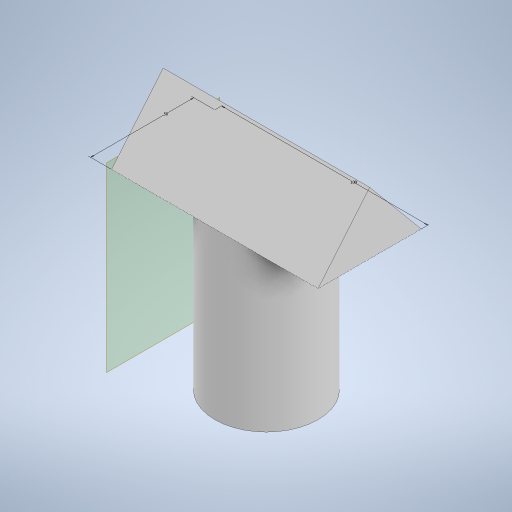
# Autodesk Inventor part: rotator_flat
Saved by Autodesk Inventor 2023.1 (Build 271208000, 208)
## iProperties
Created: 2022-10-07
Part Number: rotator_flat
Material: Generic
Document SubType Name: Modeling
Designer: swang
Density: 1 g/cm^3
Appearance: Default
Author: swang
Autodesk Inventor part; units mm, degrees
ref_plane "YZ Plane" through (0, 0, 0) normal (1, 0, 0) x (0, 1, 0)
ref_plane "XZ Plane" through (0, 0, 0) normal (0, 1, 0) x (-1, 0, 0)
ref_plane "XY Plane" through (0, 0, 0) normal (0, 0, 1) x (1, 0, 0)
sketch "Sketch1" plane through (0, 0, 0) normal (0, 1, 0) x (-1, 0, 0)
  circle A0 centre (0, 0) radius 25
  dimension "d0" = 50
  constraints: 1 centre point, 1 coincident
  measures "d0" diameter of A0
extrude "Extrusion1" add sketch "Sketch1" along normal blind 80
sketch "Sketch3" plane through (0, 80, 0) normal (0, 1, 0) x (1, 0, 0)
  line L0 (-50, -25) -> (50, -25) construction
  line L1 (50, -25) -> (50, 25) construction
  line L2 (50, 25) -> (-50, 25) construction
  line L3 (-50, 25) -> (-50, -25) construction
  line L4 (-50, -25) -> (50, 25) construction
  line L5 (50, -25) -> (-50, 25) construction
  point P0 (0, 0)
  dimension "d7" = 100
  dimension "d8" = 50
  constraints: 12 end point, 2 midpoint, 2 parallel, 1 horizontal, 1 perpendicular
  measures "d7" distance of L1.end L2.end
  measures "d8" distance of L2.end L0.start
ref_plane "Work Plane2" through (-50, 80, -25) normal (-1, 0, 0) x (0, 0, 1)
sketch "Sketch5" plane through (-50, 80, -25) normal (-1, 0, 0) x (0, 0, 1)
  line L0 (50, 0) -> (0, 0) projected
  line L1 (50, 0) -> (0, 0)
  line L2 (25, 0) -> (25, 30) construction
  line L3 (25, 30) -> (50, 0)
  line L4 (25, 30) -> (0, 0)
  point P0 (25, -80)
  dimension "d13" = 30
  constraints: 8 end point, 1 midpoint, 1 vertical
  measures "d13" distance from line of L0 L2.end
extrude "Extrusion3" add sketch "Sketch5" against normal blind 100
body "Solid1"
